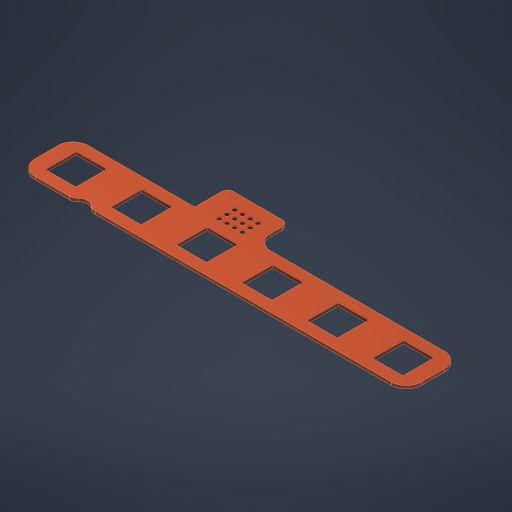
# Autodesk Inventor part: bat_contacts_v2_plate_contact
Saved by Autodesk Inventor 2024.3 (Build 283343010, 343A)
## iProperties
Created: 2025-05-07
Part Number: bat_contacts_v2_plate_contact
Material: Kupfer
Document SubType Name: Modellieren
Designer: David
Density: 8.94 g/cm^3
Appearance: Kupfer - satiniert
Sheet Metal Rule: Standard_mm
Author: David
Autodesk Inventor part; units mm, degrees
ref_plane "YZ Plane" through (0, 0, 0) normal (1, 0, 0) x (0, 1, 0)
ref_plane "XZ Plane" through (0, 0, 0) normal (0, 1, 0) x (-1, 0, 0)
ref_plane "XY Plane" through (0, 0, 0) normal (0, 0, 1) x (1, 0, 0)
sketch "Skizze1" plane through (0, 0, 0) normal (0, 0, 1) x (1, 0, 0)
  line L0 (0, 0) -> (127, 0)
  line L1 (127, 0) -> (127, 37.5)
  line L2 (127, 37.5) -> (0, 37.5)
  line L3 (0, 37.5) -> (0, 0)
  line L4 (4.75, 3.65) -> (14.75, 3.65)
  line L5 (14.75, 3.65) -> (14.75, 13.85)
  line L6 (14.75, 13.85) -> (4.75, 13.85)
  line L7 (4.75, 13.85) -> (4.75, 3.65)
  line L8 (4.75, 33.85) -> (4.75, 23.65)
  line L9 (14.75, 33.85) -> (4.75, 33.85)
  line L10 (14.75, 23.65) -> (14.75, 33.85)
  line L11 (4.75, 23.65) -> (14.75, 23.65)
  line L12 (26.25, 13.85) -> (26.25, 3.65)
  line L13 (36.25, 13.85) -> (26.25, 13.85)
  line L14 (36.25, 3.65) -> (36.25, 13.85)
  line L15 (26.25, 3.65) -> (36.25, 3.65)
  line L16 (26.25, 33.85) -> (26.25, 23.65)
  line L17 (36.25, 33.85) -> (26.25, 33.85)
  line L18 (36.25, 23.65) -> (36.25, 33.85)
  line L19 (26.25, 23.65) -> (36.25, 23.65)
  line L20 (47.75, 13.85) -> (47.75, 3.65)
  line L21 (57.75, 13.85) -> (47.75, 13.85)
  line L22 (57.75, 3.65) -> (57.75, 13.85)
  line L23 (47.75, 3.65) -> (57.75, 3.65)
  line L24 (47.75, 33.85) -> (47.75, 23.65)
  line L25 (57.75, 33.85) -> (47.75, 33.85)
  line L26 (57.75, 23.65) -> (57.75, 33.85)
  line L27 (47.75, 23.65) -> (57.75, 23.65)
  line L28 (69.25, 13.85) -> (69.25, 3.65)
  line L29 (79.25, 13.85) -> (69.25, 13.85)
  line L30 (79.25, 3.65) -> (79.25, 13.85)
  line L31 (69.25, 3.65) -> (79.25, 3.65)
  line L32 (69.25, 33.85) -> (69.25, 23.65)
  line L33 (79.25, 33.85) -> (69.25, 33.85)
  line L34 (79.25, 23.65) -> (79.25, 33.85)
  line L35 (69.25, 23.65) -> (79.25, 23.65)
  line L36 (90.75, 13.85) -> (90.75, 3.65)
  line L37 (100.75, 13.85) -> (90.75, 13.85)
  line L38 (100.75, 3.65) -> (100.75, 13.85)
  line L39 (90.75, 3.65) -> (100.75, 3.65)
  line L40 (90.75, 33.85) -> (90.75, 23.65)
  line L41 (100.75, 33.85) -> (90.75, 33.85)
  line L42 (100.75, 23.65) -> (100.75, 33.85)
  line L43 (90.75, 23.65) -> (100.75, 23.65)
  line L44 (112.25, 13.85) -> (112.25, 3.65)
  line L45 (122.25, 13.85) -> (112.25, 13.85)
  line L46 (122.25, 3.65) -> (122.25, 13.85)
  line L47 (112.25, 3.65) -> (122.25, 3.65)
  line L48 (112.25, 33.85) -> (112.25, 23.65)
  line L49 (122.25, 33.85) -> (112.25, 33.85)
  line L50 (122.25, 23.65) -> (122.25, 33.85)
  line L51 (112.25, 23.65) -> (122.25, 23.65)
  line L52 (0, 18.75) -> (40, 18.75)
  line L53 (40, 18.75) -> (40, 28.25)
  line L54 (40, 28.25) -> (60, 28.25)
  line L55 (60, 28.25) -> (60, 23.75)
  arc A0 (60, 23.75) -> (65, 18.75) centre (65, 23.75) ccw
  line L56 (65, 18.75) -> (127, 18.75)
  arc A1 (23.2272, 0) -> (17.7728, 0) centre (20.5, -1.25) ccw
  line L57 (0, 17.5) -> (40, 17.5)
  line L58 (40, 17.5) -> (40, 18.75)
  line L59 (127, 17.5) -> (65, 17.5)
  arc A2 (60, 22.5) -> (65, 17.5) centre (65, 22.5) ccw
  line L60 (60, 22.5) -> (60, 23.75)
  point P0 (63.5, 37.5)
  point P1 (42, 18.75)
  point P2 (85, 18.75)
  point P3 (63.5, 0)
  point P4 (55, 23.25)
  point P5 (52.46, 23.25)
  point P6 (49.92, 23.25)
  point P7 (47.38, 23.25)
  point P8 (55, 20.71)
  point P9 (52.46, 20.71)
  point P10 (49.92, 20.71)
  point P11 (47.38, 20.71)
  point P12 (55, 18.17)
  point P13 (52.46, 18.17)
  point P14 (49.92, 18.17)
  point P15 (47.38, 18.17)
  point P16 (31.25, 3.65)
  point P17 (4.75, 8.75)
  dimension "d0" = 127
  dimension "d1" = 37.5
  dimension "d2" = 10.2
  dimension "d3" = 10
  dimension "d6" = 20
  dimension "d9" = 21.5
  dimension "d13" = 5.75
  dimension "d17" = 43
  dimension "d18" = 21.5
  dimension "d19" = 28.25
  dimension "d20" = 60
  dimension "d21" = 5
  dimension "d22" = 20
  dimension "d24" = 5
  dimension "d36" = 2.54
  dimension "d39" = 2.54
  dimension "d43" = 3
  dimension "d44" = 1.25
  dimension "d45" = 10.75
  dimension "d48" = 8.75
  dimension "d49" = 8.75
  dimension "d50" = 5
  constraints: 122 end point, 7 perpendicular, 6 horizontal, 6 midpoint, 6 point on circle, 5 parallel, 5 point on line, 5 tangent, 3 centre point, 3 horizontal alignment, 2 vertical, 1 equal radius, 99 other
  measures "d0" distance of L1.end L2.end
  measures "d1" distance of L2.end L0.start
  measures "d2" distance of L6.end L4.start
  measures "d3" distance of L4.start L4.end
  measures "d6" distance of L6.end L8.start
  measures "d9" distance of L6.end L12.start
  measures "d13" distance from line of point (63.5, 37.5) L26
  measures "d17" distance of point (85, 18.75) point (42, 18.75)
  measures "d18" horizontal distance of point (63.5, 0) point (42, 18.75)
  measures "d19" distance between parallel lines of L0 L54
  measures "d20" distance between parallel lines of L3 L55
  measures "d21" radius of A0
  measures "d22" distance of L53.end L54.end
  measures "d24" distance from line of L55 point (55, 23.25)
  measures "d36" distance of point (55, 23.25) point (52.46, 23.25)
  measures "d39" distance of point (55, 23.25) point (55, 20.71)
  measures "d43" radius of A1
  measures "d44" distance from line of A1.centre L0
  measures "d45" horizontal distance of A1.centre point (31.25, 3.65)
  measures "d48" distance from line of point (4.75, 8.75) L57
  measures "d49" distance from line of L0 point (4.75, 8.75)
  measures "d50" distance from line of point (47.38, 23.25) L54
extrude "Extrusion1" add sketch "Skizze1" along normal blind 1 contours L3 L57 L58 L53 L54 L24 L27 L26 L55 L60 A2 L59 L1 L0 A1 | L54 L26 L27 L24
fillet "Rundung1" radius 5 2 edges at (127, 0, 0.5) (0, 0, 0.5)
hole "Bohrung1" at (55, 23.25, 0) at (55, 20.71, 0) at (52.46, 20.71, 0) at (49.92, 20.71, 0) at (49.92, 23.25, 0) at (52.46, 23.25, 0) at (55, 18.17, 0) at (52.46, 18.17, 0) at (49.92, 18.17, 0) at (47.38, 18.17, 0) at (47.38, 20.71, 0) at (47.38, 23.25, 0) direction (0, 0, 1) diameter 1.4 end through all
fillet "Rundung2" radius 2 2 edges at (60, 28.25, 0.5) (40, 28.25, 0.5)
fillet "Rundung3" radius 5 2 edges at (127, 17.5, 0.5) (0, 17.5, 0.5)
fillet "Rundung4" radius 3 2 edges at (17.7728, 0, 0.5) (23.2272, 0, 0.5)
sketch "Skizze2" plane through (0, 0, 1) normal (0, 0, 1) x (1, 0, 0)
  arc A0 (0, 5) -> (5, 0) centre (5, 5) ccw projected
  line L0 (5, 0) -> (16.2647, 0) projected
  arc A1 (122, 0) -> (127, 5) centre (122, 5) ccw projected
  line L1 (127, 5) -> (127, 12.5) projected
  line L2 (0, 12.5) -> (0, 5) projected
  line L3 (112.25, 13.85) -> (122.25, 13.85) projected
  line L4 (122.25, 13.85) -> (122.25, 3.65) projected
  line L5 (122.25, 3.65) -> (112.25, 3.65) projected
  line L6 (112.25, 3.65) -> (112.25, 13.85) projected
  line L7 (90.75, 13.85) -> (100.75, 13.85) projected
  line L8 (100.75, 13.85) -> (100.75, 3.65) projected
  line L9 (100.75, 3.65) -> (90.75, 3.65) projected
  line L10 (90.75, 3.65) -> (90.75, 13.85) projected
  line L11 (69.25, 13.85) -> (79.25, 13.85) projected
  line L12 (79.25, 13.85) -> (79.25, 3.65) projected
  line L13 (79.25, 3.65) -> (69.25, 3.65) projected
  line L14 (69.25, 3.65) -> (69.25, 13.85) projected
  line L15 (47.75, 13.85) -> (57.75, 13.85) projected
  line L16 (57.75, 13.85) -> (57.75, 3.65) projected
  line L17 (57.75, 3.65) -> (47.75, 3.65) projected
  line L18 (47.75, 3.65) -> (47.75, 13.85) projected
  line L19 (26.25, 13.85) -> (36.25, 13.85) projected
  line L20 (36.25, 13.85) -> (36.25, 3.65) projected
  line L21 (36.25, 3.65) -> (26.25, 3.65) projected
  line L22 (26.25, 3.65) -> (26.25, 13.85) projected
  line L23 (4.75, 3.65) -> (4.75, 13.85) projected
  line L24 (4.75, 13.85) -> (14.75, 13.85) projected
  line L25 (14.75, 13.85) -> (14.75, 3.65) projected
  line L26 (14.75, 3.65) -> (4.75, 3.65) projected
  line L27 (60, 22.5) -> (60, 26.25) projected
  line L28 (58, 28.25) -> (42, 28.25) projected
  line L29 (40, 26.25) -> (40, 17.5) projected
  arc A2 (60, 26.25) -> (58, 28.25) centre (58, 26.25) ccw projected
  arc A3 (42, 28.25) -> (40, 26.25) centre (42, 26.25) ccw projected
  circle A4 centre (55, 23.25) radius 0.7 projected
  arc A5 (22.6176, 0.875) -> (18.3824, 0.875) centre (20.5, -1.25) ccw projected
  line L30 (24.7353, 0) -> (122, 0) projected
  arc A6 (22.6176, 0.875) -> (24.7353, 0) centre (24.7353, 3) ccw projected
  arc A7 (16.2647, 0) -> (18.3824, 0.875) centre (16.2647, 3) ccw projected
  line L31 (122, 17.5) -> (65, 17.5) projected
  arc A8 (60, 22.5) -> (65, 17.5) centre (65, 22.5) ccw projected
  line L32 (40, 17.5) -> (5, 17.5) projected
  arc A9 (127, 12.5) -> (122, 17.5) centre (122, 12.5) ccw projected
  arc A10 (5, 17.5) -> (0, 12.5) centre (5, 12.5) ccw projected
  point P0 (0, 0)
equation "\"d13\" = -0.5 * d3 + 0.5 * d9"
equation "\"d17\" = 2 * d9"
equation "\"d18\" = 0.5 * d17"
equation "\"d45\" = 0.5 * d9"
equation "\"d49\" = d48"
equation "\"Biegeradius\" = Stärke"
equation "\"BreiteBiegungsfreistellung\" = Stärke"
equation "\"TiefeBiegungsfreistellung\" = 0.5 * Stärke"
equation "\"GrößeEckenfreistellung\" = 4 * Stärke"
equation "\"MinimalRest\" = 2 * Stärke"
equation "\"Übergangsradius\" = Biegeradius"
equation "\"JacobiRadiusGröße\" = Biegeradius"
equation "\"Abstandsgröße\" = Stärke"
equation "\"Stärke\" = 0.5"
